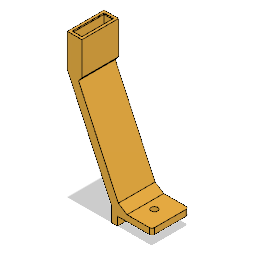
Wize_camera_mount v11 (Autodesk Fusion 360 design; units mm, degrees)
Autodesk Fusion 360 part; units mm, degrees
sketch "Sketch1" plane through (0, 0, 0) normal (0, 0, 1) x (1, 0, 0)
  line L0 (-6, 0) -> (6, 0)
  line L1 (6, 0) -> (6, -27)
  line L2 (6, -27) -> (-6, -27)
  line L3 (-6, -27) -> (-6, 0)
  line L4 (30, -105) -> (35, -105)
  line L5 (35, -105) -> (35, -117)
  line L6 (35, -117) -> (30, -117)
  line L7 (30, -117) -> (30, -105)
  line L8 (35, -105) -> (63, -105)
  line L9 (63, -105) -> (63, -110)
  line L10 (63, -110) -> (35, -110)
  line L11 (35, -110) -> (35, -105)
  line L12 (30, -105) -> (-6, -27)
  line L13 (0, 0) -> (0, -27) construction
  line L14 (6, -27) -> (3.2243, -30.2818)
  line L15 (1.7096, -27) -> (37.7096, -105)
  line L16 (42.7096, -105) -> (35.6143, -100.4602)
  dimension "d2" = 12
  dimension "d3" = 5
  dimension "d4" = 5
  dimension "d6" = 28
  dimension "d7" = 7
  dimension "d8" = 27
  dimension "d29" = 110
  dimension "d32" = 35
  dimension "d38" = 7
  dimension "d39" = 115
  dimension "d40" = 5
  dimension "d41" = 5
  constraint horizontal L0
  constraint vertical L1
  constraint horizontal L2
  constraint vertical L3
  constraint midpoint L13.start L0
  constraint horizontal L4
  constraint vertical L5
  constraint horizontal L6
  constraint vertical L7
  constraint horizontal L8
  constraint vertical L9
  constraint horizontal L10
  constraint vertical L11
  constraint coincident L2 L3.start
  constraint coincident L13.start origin
  constraint midpoint L2 L13.end
  constraint coincident L2.end L12
  constraint coincident L2 L15.start
  constraint coincident L8 L15.end
  constraint parallel L12 L15
  constraint coincident L14.end L15
  constraint coincident L8 L16.start
  constraint coincident L15 L16.end
  measures "d2" distance of L0.start L0.end
  measures "d3" distance of L5.end L6.end
  measures "d4" distance of L8.end L9.end
  measures "d6" distance of L4.end L8.end
  measures "d7" distance of L6 L10
  measures "d8" distance of L0.start L2.end
  measures "d29" distance of L0 L10
  measures "d32" distance of L4.end L13
  measures "d38" distance of L12 L15
  measures "d39" angle of L14 L15
  measures "d40" distance of L15.end L16.start
  measures "d41" distance of L15.end L16.end
extrude "Extrude1" add sketch "Sketch1" along normal blind 30
sketch "Sketch2" plane through (0, -110, 0) normal (0, -1, 0) x (-1, 0, 0)
  line L0 (-50, -30) -> (-50, 0) construction
  line L1 (-63, -15) -> (-35, -15) construction
  circle A0 centre (-50, -15) radius 2.65
  circle A1 centre (-50, -15) radius 5 construction
  line L2 (-35, 0) -> (-63, 0)
  line L3 (-63, 0) -> (-63, -30)
  line L4 (-63, -30) -> (-35, -30)
  line L5 (-35, -30) -> (-35, 0)
  dimension "d15" = 5.3
  dimension "d16" = 10
  dimension "d43" = 15
  constraint coincident L0 A0.centre
  constraint concentric A0 A1
  constraint coincident L0.start L4
  constraint coincident L0.end L2
  constraint perpendicular L0 L2
  constraint midpoint L1.start L3
  constraint midpoint L1.end L5
  constraint coincident L1 A0.centre
  measures "d15" diameter of A0
  measures "d16" diameter of A1
  measures "d43" distance of L0 L5
extrude "Extrude2" cut sketch "Sketch2" against normal through all contours A0
sketch "Sketch3" plane through (0, 0, 0) normal (0, 1, 0) x (-1, 0, 0)
  line L0 (-6, 0) -> (6, 0)
  line L1 (6, 0) -> (6, 30)
  line L2 (6, 30) -> (-6, 30)
  line L3 (-6, 30) -> (-6, 0)
  line L4 (0, 0) -> (0, 30) construction
  line L5 (-3.4, 27.375) -> (3.4, 27.375)
  line L6 (3.4, 27.375) -> (3.4, 2.625)
  line L7 (3.4, 2.625) -> (-3.4, 2.625)
  line L8 (-3.4, 2.625) -> (-3.4, 27.375)
  line L9 (-3.4, 27.375) -> (3.4, 2.625) construction
  line L10 (3.4, 27.375) -> (-3.4, 2.625) construction
  point P0 (0, 15)
  point P1 (0, 15)
  dimension "d21" = 24.75
  dimension "d22" = 6.8
  constraint coincident L4.start origin
  constraint midpoint L2 L4.end
  constraint midpoint L4 P1
  constraint perpendicular L5 L6
  constraint parallel L5 L7
  constraint parallel L6 L8
  constraint horizontal L5
  constraint coincident L9 P1
  constraint coincident L10 P1
  constraint coincident P1 P0
  measures "d21" distance of L5.end L6.end
  measures "d22" distance of L5.start L5.end
extrude "Extrude3" cut sketch "Sketch3" against normal blind 26 contours L5 L6 L7 L8
chamfer "Chamfer2" distance 0.5 angle 45 4 edges at (0, 0, 2.625) (3.4, 0, 15) (0, 0, 27.375) (-3.4, 0, 15)
fillet "Fillet1" radius 2 2 edges at (63, -107.5, 0) (63, -107.5, 30)
equation "d41 = d40"
